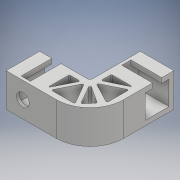
# Autodesk Inventor part: OuterFrame
Saved by Autodesk Inventor 2017 (Build 210142000, 142)
## iProperties
Created: 2017-01-06
Part Number: OuterFrame
Material: Generic
Document SubType Name: Modeling
Designer: kurti
Density: 1 g/cm^3
Appearance: Default
Author: kurti
Autodesk Inventor part; units mm, degrees
ref_plane "YZ Plane" through (0, 0, 0) normal (1, 0, 0) x (0, 1, 0)
ref_plane "XZ Plane" through (0, 0, 0) normal (0, 1, 0) x (-1, 0, 0)
ref_plane "XY Plane" through (0, 0, 0) normal (0, 0, 1) x (1, 0, 0)
sketch "Sketch1" plane through (0, 0, 0) normal (0, 0, 1) x (1, 0, 0)
  line L0 (0, 0) -> (150, 0)
  line L1 (150, 0) -> (150, 45)
  line L2 (90, 60) -> (0, 60)
  line L3 (0, 60) -> (0, 0)
  line L4 (90, 60) -> (90, 150)
  line L5 (90, 150) -> (150, 150)
  line L6 (150, 150) -> (150, 45)
  dimension "d5" = 90
  dimension "d6" = 60
  dimension "d7" = 90
  dimension "d9" = 60
  dimension "d10" = 150
  dimension "d11" = 150
  constraints: 14 end point, 3 parallel, 1 horizontal, 1 perpendicular
  measures "d5" distance of L2.start L2.end
  measures "d6" distance of L2.end L0.start
  measures "d7" distance of L2.start L4.end
  measures "d9" distance of L4.end L5.end
  measures "d10" distance of L0.start L0.end
  measures "d11" distance between parallel lines of L5 L0
extrude "Extrusion1" add sketch "Sketch1" along normal blind 60
sketch "Sketch2" plane through (0, 60, 0) normal (0, 1, 0) x (1, 0, 0)
  line L0 (0, 0) -> (150, 0) construction
  line L1 (0, 0) -> (60, -60) construction
  line L2 (0, 0) -> (84.8528, 0) construction
  line L3 (8.75, -51.25) -> (8.75, -8.75)
  line L4 (8.75, -8.75) -> (51.25, -8.75)
  line L5 (51.25, -8.75) -> (51.25, -51.25)
  line L6 (51.25, -51.25) -> (8.75, -8.75) construction
  line L7 (8.75, -51.25) -> (51.25, -8.75) construction
  line L8 (30, -30) -> (30, -51.25) construction
  line L9 (30, -51.25) -> (21.75, -51.25) construction
  line L10 (30, -51.25) -> (38.25, -51.25) construction
  line L11 (21.75, -51.25) -> (21.75, -60)
  line L12 (0, -60) -> (150, -60) projected
  line L13 (38.25, -51.25) -> (38.25, -60)
  line L14 (21.75, -60) -> (38.25, -60)
  line L15 (51.25, -51.25) -> (38.25, -51.25)
  line L16 (21.75, -51.25) -> (8.75, -51.25)
  dimension "d14" = 84.8528
  dimension "d15" = 45
  dimension "d16" = 42.5
  dimension "d17" = 42.5
  dimension "d32" = 8.25
  dimension "d33" = 8.25
  dimension "d34" = 90
  constraints: 30 end point, 5 parallel, 4 perpendicular, 3 horizontal, 3 midpoint, 2 point on line, 1 equal length, 1 vertical
  measures "d14" distance of L0.start L1.end
  measures "d15" angle of L1 L2
  measures "d16" distance of L3.end L4.end
  measures "d17" distance of L3.start L3.end
  measures "d32" distance of L8.end L9.end
  measures "d33" distance of L10.end L8.end
  measures "d34" angle of L10 L5
extrude "Extrusion2" cut sketch "Sketch2" against normal blind 55
sketch "Sketch4" plane through (150, 0, 0) normal (1, 0, 0) x (0, 0, -1)
  line L0 (0, 150) -> (0, 60) construction
  line L1 (0, 150) -> (-60, 90) construction
  line L2 (0, 150) -> (84.8528, 150) construction
  line L3 (-51.25, 98.75) -> (-8.75, 98.75)
  line L4 (-8.75, 98.75) -> (-8.75, 141.25)
  line L5 (-8.75, 141.25) -> (-51.25, 141.25)
  line L6 (-51.25, 98.75) -> (-8.75, 141.25) construction
  line L7 (-8.75, 98.75) -> (-51.25, 141.25) construction
  line L8 (-30, 120) -> (-60, 120) construction
  line L9 (-60, 120) -> (-60, 128.25)
  line L10 (-60, 0) -> (-60, 150) projected
  line L11 (-60, 128.25) -> (-51.25, 128.25)
  line L12 (-60, 120) -> (-60, 111.75)
  line L13 (-60, 111.75) -> (-51.25, 111.75)
  line L14 (-51.25, 141.25) -> (-51.25, 128.25)
  line L15 (-51.25, 111.75) -> (-51.25, 98.75)
  point P0 (0, 0)
  dimension "d26" = 84.8528
  dimension "d27" = 135
  dimension "d28" = 42.5
  dimension "d29" = 42.5
  dimension "d35" = 8.25
  dimension "d36" = 8.25
  dimension "d37" = 90
  constraints: 28 end point, 6 perpendicular, 3 horizontal, 3 midpoint, 3 parallel, 2 point on line, 1 equal length
  measures "d26" distance of L0.start L1.end
  measures "d27" angle of L1 L2
  measures "d28" distance of L5.end L4.end
  measures "d29" distance of L4.end L3.end
  measures "d35" distance of L8.end L9.end
  measures "d36" distance of L8.end L12.end
  measures "d37" angle of L9 L2
extrude "Extrusion4" cut sketch "Sketch4" against normal blind 55
hole "Hole2" at (30, 5, 30) direction (0, -1, 0) diameter 22.5 end through all
hole "Hole4" at (95, 120, 30) direction (-1, 0, 0) diameter 22.5 end through all
fillet "Fillet1" radius 5 1 edges at (90, 60, 30)
fillet "Fillet2" radius 60 1 edges at (150, 0, 30)
sketch "Sketch5" plane through (0, 0, 60) normal (0, 0, 1) x (1, 0, 0)
  line L0 (0, 0) -> (90, 0) construction
  line L1 (0, 0) -> (60, 0) construction
  line L2 (60, 0) -> (60, 60) construction
  line L3 (60, 60) -> (0, 60) construction
  line L4 (0, 60) -> (0, 0) construction
  line L5 (149.6513, 150.4559) -> (89.6513, 150.4559) construction
  line L6 (89.6513, 150.4559) -> (89.6513, 90.4559) construction
  line L7 (89.6513, 90.4559) -> (149.6513, 90.4559) construction
  line L8 (149.6513, 90.4559) -> (149.6513, 150.4559) construction
  line L9 (89.6513, 90.4559) -> (149.6513, 90.4559) construction
  line L10 (149.6513, 90.4559) -> (149.6513, 80.4559) construction
  line L11 (149.6513, 80.4559) -> (89.6513, 80.4559) construction
  line L12 (89.6513, 80.4559) -> (89.6513, 90.4559) construction
  line L13 (60, 60) -> (70, 60) construction
  line L14 (70, 60) -> (70, 0) construction
  line L15 (70, 0) -> (60, 0) construction
  line L16 (60, 0) -> (60, 60) construction
  line L17 (70, 60) -> (89.6513, 60) construction
  line L18 (89.6513, 60) -> (89.6513, 80.4559) construction
  line L19 (89.6513, 80.4559) -> (70, 80.4559) construction
  line L20 (70, 80.4559) -> (70, 60) construction
  line L21 (70, 60) -> (90, 60) construction
  line L22 (90, 60) -> (90, 50) construction
  line L23 (90, 50) -> (70, 50) construction
  line L24 (70, 50) -> (70, 60) construction
  line L25 (90, 50) -> (100, 50) construction
  line L26 (100, 50) -> (100, 60.8297) construction
  line L27 (100, 60.8297) -> (90, 60.8297) construction
  line L28 (90, 60.8297) -> (90, 50) construction
  line L29 (100, 60.8297) -> (89.6513, 60.8297) construction
  line L30 (89.6513, 60.8297) -> (89.6513, 80.4559) construction
  line L31 (89.6513, 80.4559) -> (100, 80.4559) construction
  line L32 (100, 80.4559) -> (100, 60.8297) construction
  line L33 (149.6513, 80.4559) -> (139.6513, 80.4559) construction
  line L34 (139.6513, 80.4559) -> (139.6513, 0.4559) construction
  line L35 (139.6513, 0.4559) -> (149.6513, 0.4559) construction
  line L36 (149.6513, 0.4559) -> (149.6513, 80.4559) construction
  line L37 (70, 0) -> (139.6513, 0) construction
  line L38 (139.6513, 0) -> (139.6513, 10) construction
  line L39 (139.6513, 10) -> (70, 10) construction
  line L40 (70, 10) -> (70, 0) construction
  arc A0 (90, 0) -> (150, 60) centre (90, 60) ccw construction
  line L41 (123.1662, 10) -> (113.1662, 10) construction
  line L42 (113.1662, 10) -> (113.1662, 20) construction
  line L43 (113.1662, 20) -> (123.1662, 20) construction
  line L44 (123.1662, 20) -> (123.1662, 10) construction
  line L45 (123.1662, 20) -> (133.1662, 20) construction
  line L46 (133.1662, 20) -> (133.1662, 30) construction
  line L47 (133.1662, 30) -> (123.1662, 30) construction
  line L48 (123.1662, 30) -> (123.1662, 20) construction
  line L49 (133.1662, 30) -> (143.1662, 30) construction
  line L50 (143.1662, 30) -> (143.1662, 40) construction
  line L51 (143.1662, 40) -> (133.1662, 40) construction
  line L52 (133.1662, 40) -> (133.1662, 30) construction
  line L53 (70, 10) -> (90, 50)
  line L54 (113.1662, 10) -> (90, 50)
  line L55 (70, 10) -> (113.1662, 10)
  line L56 (100, 60.8297) -> (139.6513, 40)
  line L57 (100, 60.8297) -> (139.6513, 80.4559)
  line L58 (139.6513, 40) -> (139.6513, 80.4559)
  line L59 (113.1662, 10) -> (139.6513, 40) construction
  line L60 (90, 50) -> (100, 60.8297) construction
  line L61 (95, 55.4149) -> (117.8355, 15.289)
  line L62 (95, 55.4149) -> (131.9763, 31.3064)
  line L63 (117.8355, 15.289) -> (131.9763, 31.3064)
  line L64 (90, 50) -> (83, 50) construction
  line L65 (83, 50) -> (63.0073, 10)
  line L66 (63.0073, 10) -> (63.0073, 50)
  line L67 (63.0073, 50) -> (83, 50)
  line L68 (100, 69.1023) -> (139.6513, 88.1548)
  line L69 (139.6513, 88.1548) -> (100, 88.1548)
  line L70 (100, 88.1548) -> (100, 69.1023)
  dimension "d76" = 60
  dimension "d77" = 60
  dimension "d78" = 60
  dimension "d79" = 60
  dimension "d80" = 60
  dimension "d81" = 10
  dimension "d82" = 10
  dimension "d83" = 60
  dimension "d84" = 10
  dimension "d85" = 10
  dimension "d86" = 10
  dimension "d87" = 80
  dimension "d88" = 10
  dimension "d89" = 10
  dimension "d90" = 10
  dimension "d91" = 10
  dimension "d92" = 10
  dimension "d93" = 10
  dimension "d94" = 10
  dimension "d97" = 7
  constraints: 140 end point, 28 parallel, 14 perpendicular, 13 horizontal, 7 point on line, 4 collinear, 1 midpoint, 1 point on circle
  measures "d76" distance of L3.end L2.end
  measures "d77" distance of L2.end L1.end
  measures "d78" distance of L7.end L6.end
  measures "d79" distance of L6.end L5.end
  measures "d80" distance of L10.end L11.end
  measures "d81" distance of L9.end L10.end
  measures "d82" distance of L14.end L15.end
  measures "d83" distance of L13.end L14.end
  measures "d84" distance of L21.end L22.end
  measures "d85" distance of L27.end L26.end
  measures "d86" distance of L35.end L34.end
  measures "d87" distance of L34.end L33.end
  measures "d88" distance of L38.end L37.end
  measures "d89" distance of L42.end L43.end
  measures "d90" distance of L41.end L42.end
  measures "d91" distance of L47.end L46.end
  measures "d92" distance of L46.end L45.end
  measures "d93" distance of L51.end L50.end
  measures "d94" distance of L50.end L49.end
  measures "d97" distance of L22.end L64.end
extrude "Extrusion5" cut sketch "Sketch5" against normal blind 94
fillet "Fillet3" radius 2 13 edges at (113.1662, 10, 30) (131.9763, 31.3064, 30) (117.8355, 15.289, 30) (70, 10, 30) (63.0073, 50, 30) (83, 50, 30) (90, 50, 30) (95, 55.4149, 30) (100, 60.8297, 30) (100, 69.1023, 30) (100, 88.1548, 30) (139.6513, 80.4559, 30) (139.6513, 40, 30)
fillet "Fillet4" radius 1 2 edges at (63.0073, 10, 30) (139.6513, 88.1548, 30)
body "Solid1"
